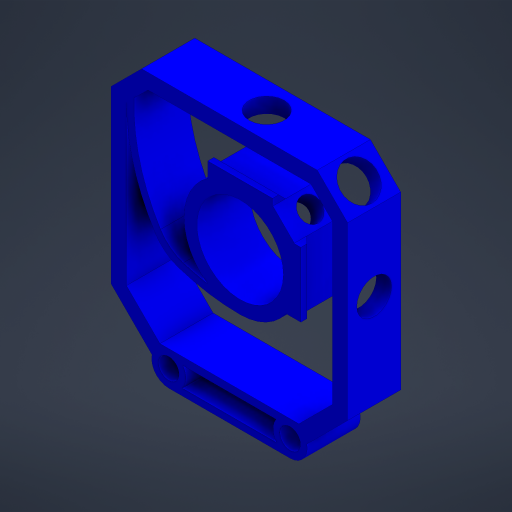
# Autodesk Inventor part: Laser Holder (Battery Pointer)
Saved by Autodesk Inventor 2023.4 (Build 274418000, 418)
## iProperties
Created: 2022-07-25
Part Number: Laser Holder (Battery Pointer)
Material: Generic
Document SubType Name: Modeling
Designer: xSibe
Density: 1 g/cm^3
Appearance: Plastic Blue
Author: xSibe
Autodesk Inventor part; units mm, degrees
ref_plane "YZ Plane" through (0, 0, 0) normal (1, 0, 0) x (0, 1, 0)
ref_plane "XZ Plane" through (0, 0, 0) normal (0, 1, 0) x (-1, 0, 0)
sketch "Sketch1" plane through (0, 0, 0) normal (0, 0, 1) x (1, 0, 0)
  line L0 (149.6, 24.9) -> (151.367767, 26.667767)
  line L1 (149.6, 24.9) -> (152.1, 24.9) construction
  circle A0 centre (151.367767, 26.667767) radius 7.125
  circle A1 centre (151.367767, 26.667767) radius 6.45
  circle A2 centre (151.367767, 26.667767) radius 9.25
  line L2 (151.367767, 26.667767) -> (151.367767, 35.917767)
  line L3 (151.367767, 35.917767) -> (151.367767, 35.417767)
  line L4 (146.030267, 34.167767) -> (156.705267, 34.167767)
  line L5 (156.705267, 34.167767) -> (156.705267, 36.667767)
  line L6 (156.705267, 36.667767) -> (146.030267, 36.667767)
  line L7 (146.030267, 36.667767) -> (146.030267, 34.167767)
  line L8 (146.030267, 34.167767) -> (156.705267, 36.667767) construction
  line L9 (156.705267, 34.167767) -> (146.030267, 36.667767) construction
  line L10 (151.367767, 26.667767) -> (157.908505, 33.208505)
  line L11 (157.908505, 33.208505) -> (157.466563, 32.766563)
  line L12 (160.29499, 32.059456) -> (156.759456, 35.59499)
  line L13 (156.759456, 35.59499) -> (154.638136, 33.47367)
  line L14 (154.638136, 33.47367) -> (158.17367, 29.938136)
  line L15 (158.17367, 29.938136) -> (160.29499, 32.059456)
  line L16 (160.29499, 32.059456) -> (154.638136, 33.47367) construction
  line L17 (156.759456, 35.59499) -> (158.17367, 29.938136) construction
  line L18 (160.29499, 32.059456) -> (165.29499, 32.059456) construction
  line L19 (158.867767, 21.330267) -> (158.867767, 32.005267)
  line L20 (158.867767, 32.005267) -> (161.367767, 32.005267)
  line L21 (161.367767, 32.005267) -> (161.367767, 21.330267)
  line L22 (161.367767, 21.330267) -> (158.867767, 21.330267)
  line L23 (151.367767, 35.917767) -> (151.367767, 37.917767)
  line L24 (161.367767, 26.667767) -> (163.367767, 26.667767)
  line L25 (139.382233, 5.432233) -> (159.817767, 5.432233)
  line L26 (169.067767, 14.682233) -> (169.067767, 39.367767)
  line L27 (164.067767, 44.367767) -> (135.132233, 44.367767)
  line L28 (130.132233, 39.367767) -> (130.132233, 14.682233)
  line L29 (130.132233, 5.432233) -> (169.067767, 44.367767) construction
  line L30 (169.067767, 5.432233) -> (130.132233, 44.367767) construction
  line L31 (139.382233, 5.432233) -> (130.132233, 14.682233)
  line L32 (159.817767, 5.432233) -> (169.067767, 14.682233)
  line L33 (164.067767, 44.367767) -> (169.067767, 39.367767)
  line L34 (135.132233, 44.367767) -> (130.132233, 39.367767)
  line L35 (134.096699, 46.867767) -> (127.632233, 40.403301)
  line L36 (127.632233, 40.403301) -> (127.632233, 13.646699)
  line L37 (127.632233, 13.646699) -> (138.346699, 2.932233)
  line L38 (138.346699, 2.932233) -> (160.853301, 2.932233)
  line L39 (160.853301, 2.932233) -> (171.567767, 13.646699)
  line L40 (171.567767, 13.646699) -> (171.567767, 40.403301)
  line L41 (171.567767, 40.403301) -> (165.103301, 46.867767)
  line L42 (165.103301, 46.867767) -> (134.096699, 46.867767)
  line L43 (136.167767, 41.867767) -> (132.632233, 38.332233)
  line L44 (132.632233, 38.332233) -> (132.632233, 15.717767)
  line L45 (132.632233, 15.717767) -> (140.417767, 7.932233)
  line L46 (140.417767, 7.932233) -> (158.782233, 7.932233)
  line L47 (158.782233, 7.932233) -> (166.567767, 15.717767)
  line L48 (166.567767, 15.717767) -> (166.567767, 38.332233)
  line L49 (166.567767, 38.332233) -> (163.032233, 41.867767)
  line L50 (163.032233, 41.867767) -> (136.167767, 41.867767)
  line L51 (166.567767, 15.717767) -> (166.567767, 12.182233)
  line L52 (132.632233, 15.717767) -> (132.632233, 12.182233)
  line L53 (130.132233, 14.682233) -> (130.132233, 11.146699)
  line L54 (169.067767, 14.682233) -> (169.067767, 11.146699)
  line L55 (151.367767, 17.417767) -> (138.867767, 17.417767)
  line L56 (138.867767, 17.417767) -> (138.867767, 19.917767)
  arc A3 (138.867767, 19.917767) -> (151.367767, 17.417767) centre (151.367767, 49.917767) ccw
  arc A4 (132.632233, 38.332233) -> (138.867767, 19.917767) centre (162.940339, 38.332233) ccw
  arc A5 (139.658715, 20.94432) -> (146.004295, 19.131477) centre (151.367767, 49.917767) ccw
  arc A6 (133.910356, 39.610356) -> (139.658715, 20.94432) centre (162.940339, 38.332233) ccw
  line L57 (139.658715, 20.94432) -> (138.250304, 23.009842)
  line L58 (138.867767, 19.917767) -> (137.432015, 21.964378)
  arc A7 (137.432015, 21.964378) -> (141.186567, 19.053659) centre (143.412637, 25.801947) ccw
  arc A8 (138.250304, 23.009842) -> (141.987033, 20.108971) centre (144.028372, 26.595653) ccw
  line L59 (132.55, 7.7) -> (132.55, 42.1)
  line L60 (166.65, 7.7) -> (166.65, 42.1)
  line L61 (132.55, 24.9) -> (166.65, 24.9)
  circle A9 centre (139.6, 3.85) radius 1.5625
  circle A10 centre (159.6, 3.85) radius 1.5625
  circle A11 centre (139.6, 3.85) radius 2.8125
  circle A12 centre (159.6, 3.85) radius 2.8125
  circle A13 centre (159.6, 3.85) radius 1.705
  circle A14 centre (139.6, 3.85) radius 1.705
  line L62 (138.151966, 6.6625) -> (161.048034, 6.6625)
  line L63 (139.6, 1.0375) -> (159.6, 1.0375)
  line L64 (139.6, 5.555) -> (159.6, 5.555)
  line L65 (139.6, 2.145) -> (159.6, 2.145)
  point P0 (146.030267, 34.222474)
  point P1 (158.922474, 21.330267)
  point P2 (158.922474, 32.005267)
  point P3 (159.432855, 31.197321)
  point P4 (155.897321, 34.732855)
  point P5 (156.705267, 34.222474)
  point P6 (155.332233, 34.167767)
  point P7 (146.201772, 33.417767)
  point P8 (158.117767, 21.501772)
  point P9 (158.867767, 30.632233)
  point P10 (10.892767, 26.667767)
  point P11 (160.172403, 32.005267)
  point P12 (158.117767, 31.833762)
  point P13 (156.533762, 33.417767)
  point P14 (1.767767, 35.792767)
  point P15 (156.705267, 35.472403)
  point P16 (8.220116, 33.120116)
  point P17 (166.567767, 12.182233)
  point P18 (137.768638, 21.484534)
  point P19 (138.579906, 22.52646)
  point P20 (156.705267, 35.540801)
  point P21 (160.240801, 32.005267)
  point P22 (8.717767, 27.502932)
  point P23 (158.335441, 2.932233)
  point P24 (160.89125, 2.970183)
  point P25 (132.632233, 24.9)
  point P26 (135.771305, 24.9)
  point P27 (136.848125, 4.430808)
  point P28 (141.92523, 5.432233)
  point P29 (157.27477, 5.432233)
  point P30 (162.351875, 4.430808)
  point P31 (141.836768, 2.145)
  point P32 (141.836768, 5.555)
  point P33 (157.363232, 5.555)
  point P34 (157.363232, 2.145)
  dimension "d2" = 2.5
  dimension "d3" = 45
  dimension "d4" = 14.25
  dimension "d5" = 0.675
  dimension "d6" = 2.125
  dimension "d7" = 0.5
  dimension "d8" = 10.675
  dimension "d9" = 2.5
  dimension "d10" = 0.625
  dimension "d11" = 5
  dimension "d12" = 135
  dimension "d13" = 3
  dimension "d14" = 2
  dimension "d15" = 2
  dimension "d16" = 38.93553
  dimension "d17" = 38.93553
  dimension "d18" = 9.25
  dimension "d19" = 9.25
  dimension "d20" = 9.25
  dimension "d21" = 9.25
  dimension "d22" = 5
  dimension "d23" = 5
  dimension "d24" = 5
  dimension "d25" = 5
  dimension "d26" = 2.5
  dimension "d46" = 2.5
  dimension "d50" = 12.5
  dimension "d51" = 2.5
  dimension "d52" = 1.25
  dimension "d53" = 2.5
  dimension "d54" = 2.5
  dimension "d61" = 1.25
  dimension "d62" = 1.25
  dimension "d63" = 0.1425
  dimension "d64" = 0.1425
  constraints: 128 end point, 24 point on circle, 18 point on line, 13 parallel, 11 centre point, 11 tangent, 10 horizontal, 10 midpoint, 8 perpendicular, 4 symmetric about line, 2 equal length, 2 vertical, 1 coincident, 21 other
  measures "d2" distance of L0.start L0.end
  measures "d3" angle of L1 L0
  measures "d4" diameter of A0
  measures "d5" radial gap between concentric circles of A0 A1
  measures "d6" radial gap between concentric circles of A0 A2
  measures "d7" distance of L2.end L3.end
  measures "d8" distance of L6.end L5.end
  measures "d9" distance of L5.end L4.end
  measures "d10" distance of L10.end L11.end
  measures "d11" distance of L12.start L12.end
  measures "d12" angle of L18 L12
  measures "d13" distance of L13.end L12.end
  measures "d14" distance of L2.end L23.end
  measures "d15" distance of L24.start L24.end
  measures "d16" distance of L29.end L30.end
  measures "d17" distance of L30.end L29.start
  measures "d18" distance of L25.start L29.start
  measures "d19" distance of L28.end L29.start
  measures "d20" distance of L25.end L30.start
  measures "d21" distance of L26.start L30.start
  measures "d22" distance of L27.start L29.end
  measures "d23" distance of L26.end L29.end
  measures "d24" distance of L27.end L30.end
  measures "d25" distance of L28.start L30.end
  measures "d26" distance between parallel lines of L27 L42
  measures "d46" distance between parallel lines of L27 L50
  measures "d50" distance of L55.start L55.end
  measures "d51" distance of L55.end L56.end
  measures "d52" radial gap between concentric circles of A3 A5
  measures "d53" distance of L57.start L57.end
  measures "d54" distance of L56.end L58.end
  measures "d63" radial gap between concentric circles of A10 A13
  measures "d64" radial gap between concentric circles of A9 A14
extrude "Extrusion1" add sketch "Sketch1" along normal mid plane 8.75 contours L61 A2 L7 L4 L2 A0 | A0 L61 L19 L22 A2 | A0 L14 L15 L19 L61 | L2 L4 L13 L14 A0 | L14 L13 L4 L5 A2 L10 | L10 A2 L20 L19 L15 L14 | L61 A2 L22 L19 | L19 L15 A2 L61 | L4 L7 A2 L2 | L2 A2 L13 L4 | L7 L6 L23 A2 | A2 A3 A7 L58 A4 L61 A6 A5 | L61 A4 L43 A6 | L19 L20 A2 L15 | L61 L21 L22 A2 | A2 L15 L20 L21 L61 | L13 A2 L5 L4 | A2 L5 L13 L12 L15 L20 | L23 L6 L5 L13 A2 | A5 L57 A8 | L43 L44 L61 L59 L34 L27 L33 L60 L48 L49 L50 | A8 L57 A6 | A2 L20 L15 | L13 L5 A2 | L58 A7 | L44 L52 L31 L59 L61 | L61 L60 L32 L51 L48 | L59 L31 L28 L34 | L60 L33 L26 L32 | L31 A11 L37 L59 | L59 L37 L53 L31 | L32 L60 L39 A12 | L32 L54 L39 L60 | L62 A11 L31 | L32 A12 L62 | A11 L64 A14 L31 | L31 A14 L37 A11 | L62 A12 L64 A11 | L37 A14 L65 A11 | A12 L39 A13 L32 | L32 A13 L64 A12 | A12 L65 A13 L39 | L64 A12 L25 A11 | A11 L25 A14 L64 | A11 L65 A12 L63 | L64 A13 L25 A12 | A11 L38 A14 L25 | A14 L38 A11 L65 | L25 A13 L38 A12 | L65 A12 L38 A13
sketch "Sketch2" plane through (0, 0, 0) normal (0, 0, 1) x (1, 0, 0)
  circle A0 centre (151.367767, 26.667767) radius 7.125
  circle A1 centre (151.367767, 26.667767) radius 6.25
  line L0 (130.132233, 11.146699) -> (136.848125, 4.430808)
  line L1 (162.351875, 4.430808) -> (169.067767, 11.146699)
  line L2 (139.6, 1.0375) -> (159.6, 1.0375)
  arc A2 (141.836768, 2.145) -> (141.92523, 5.432233) centre (139.6, 3.85) ccw
  arc A3 (157.27477, 5.432233) -> (157.363232, 2.145) centre (159.6, 3.85) ccw
  line L3 (169.067767, 11.146699) -> (169.067767, 39.367767)
  line L4 (169.067767, 39.367767) -> (164.067767, 44.367767)
  line L5 (164.067767, 44.367767) -> (135.132233, 44.367767)
  line L6 (135.132233, 44.367767) -> (130.132233, 39.367767)
  line L7 (130.132233, 39.367767) -> (130.132233, 11.146699)
  arc A4 (159.6, 1.0375) -> (162.351875, 4.430808) centre (159.6, 3.85) ccw
  arc A5 (136.848125, 4.430808) -> (139.6, 1.0375) centre (139.6, 3.85) ccw
  line L8 (141.92523, 5.432233) -> (157.27477, 5.432233)
  line L9 (157.363232, 2.145) -> (141.836768, 2.145)
  point P0 (0, 0)
  point P1 (158.492767, 26.667767)
  point P2 (158.492767, 26.667767)
  point P3 (8.767767, 26.667767)
  dimension "d30" = 0.875
  constraints: 1 centre point, 1 other
extrude "Extrusion2" [suppressed]
sketch "Sketch3" plane through (161.367767, 13.646699, -4.375) normal (1, 0, 0) x (0, 0, -1)
  line L0 (0, 7.683568) -> (-8.75, 7.683568)
  line L1 (0, 18.358568) -> (0, 7.683568)
  line L2 (0, 18.358568) -> (-8.75, 18.358568)
  line L3 (-8.75, 7.683568) -> (-8.75, 18.358568)
  line L4 (-4.375, 18.358568) -> (-4.375, 7.683568)
  circle A0 centre (-4.375, 13.021068) radius 2.875
  point P0 (-4.375, -13.646699)
  dimension "d33" = 5.75
  constraints: 3 midpoint, 2 end point, 1 centre point
  measures "d33" diameter of A0
extrude "Extrusion3" cut sketch "Sketch3" along normal up to surface (7.7 mm away) contours A0 L4 | L4 A0
sketch "Sketch4" plane through (160.763322, 32.005267, -4.375) normal (0, 1, 0) x (1, 0, 0)
  line L0 (0.604445, 0) -> (0.604445, -8.75)
  line L1 (-0.522521, 0) -> (0.604445, 0)
  line L2 (0.604445, -8.75) -> (-0.522521, -8.75)
  line L3 (0.604445, -8.75) -> (-0.46592, -8.75)
  line L4 (-0.46592, -8.75) -> (-0.46592, -7.75)
  line L5 (-0.46592, -7.75) -> (0.604445, -7.75)
  line L6 (0.604445, -7.75) -> (0.604445, -8.75)
  line L7 (0.604445, -7.75) -> (-0.522521, -6.623034)
  line L8 (0.604445, -7.75) -> (2.198216, -7.75) construction
  line L9 (-0.522521, -4.375) -> (0.604445, -4.375)
  line L10 (0.604445, -1) -> (-0.522521, -2.126966)
  line L11 (-0.522521, 0) -> (-0.522521, -8.75)
  point P0 (-160.763322, -4.375)
  point P1 (0.604445, -1)
  point P2 (0.604445, -7.75)
  point P3 (0.604445, -7.75)
  dimension "d36" = 1
  dimension "d37" = 135
  constraints: 16 end point, 3 horizontal, 2 midpoint, 2 parallel, 2 symmetric about line, 1 equal length, 1 perpendicular, 1 point on line
  measures "d36" distance of L3.end L4.end
  measures "d37" angle of L8 L7
extrude "Extrusion4" cut sketch "Sketch4" against normal up to surface (10.675 mm away) contours L0 L9 L11 L10 | L0 L7 L11 L9
ref_plane "Work Plane1" through (161.367767, 36.667767, 4.375) normal (0.7071068, -0.7071068, 0) x (0, 0, -1)
mirror "Mirror1" about plane through (161.367767, 36.667767, 4.375) normal (0.7071068, -0.7071068, 0) of "Extrusion3", "Extrusion4"
sketch "Sketch5" plane through (95, 113.435534, 4.375) normal (0.7071068, 0.7071068, 0) x (0.7071068, -0.7071068, 0)
  line L0 (98.712107, 8.75) -> (103.712107, 8.75)
  line L1 (103.712107, 0) -> (98.712107, 0)
  circle A0 centre (101.212107, 4.375) radius 1.875
  line L2 (103.663742, 4.375) -> (98.760472, 4.375)
  circle A1 centre (101.212107, 4.375) radius 3
  line L3 (98.712107, 8.75) -> (98.712107, 0)
  line L4 (103.712107, 8.75) -> (103.712107, 0)
  dimension "d40" = 3.75
  dimension "d41" = 6
  constraints: 2 centre point, 2 end point, 1 coincident, 1 midpoint
  measures "d40" diameter of A0
  measures "d41" diameter of A1
extrude "Extrusion5" cut sketch "Sketch5" against normal blind 5 contours L3 A1 | A1 L4 L3 | A1 L4 | L2 A0 | A0 L2
extrude "Extrusion6" cut sketch "Sketch5" against normal up to next from surface at -11.371046 contours L2 A0 | A0 L2
equation "\"d19\" = d18"
equation "\"d20\" = d18"
equation "\"d21\" = d20"
equation "\"d23\" = d22"
equation "\"d24\" = d22"
equation "\"d25\" = d24"
body "Solid1"
